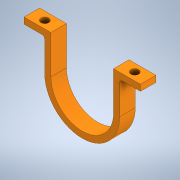
# Autodesk Inventor part: motor_support_v2
Saved by Autodesk Inventor 2020.3 (Build 243373000, 373)
## iProperties
Created: 2020-06-21
Part Number: motor_support_v2
Material: PET Plastic
Document SubType Name: Modeling
Designer: Devin
Density: 1.541 g/cm^3
Appearance: Orange
Author: Devin
Autodesk Inventor part; units mm, degrees
ref_plane "YZ Plane" through (0, 0, 0) normal (1, 0, 0) x (0, 1, 0)
ref_plane "XZ Plane" through (0, 0, 0) normal (0, 1, 0) x (-1, 0, 0)
ref_plane "XY Plane" through (0, 0, 0) normal (0, 0, 1) x (1, 0, 0)
sketch "Sketch1" plane through (0, 0, 0) normal (0, 0, 1) x (1, 0, 0)
  line L0 (-22.529, 12.5) -> (-14.529, 12.5)
  line L1 (22.5896, 12.5) -> (14.571, 12.5)
  line L2 (12.171, 14.9) -> (22.5896, 14.9)
  line L3 (22.5896, 14.9) -> (22.5896, 12.5)
  line L4 (-12.129, 14.9) -> (-22.529, 14.9)
  line L5 (-22.529, 14.9) -> (-22.529, 12.5)
  line L6 (-12.129, 0) -> (-12.129, 14.9)
  line L7 (12.171, 0) -> (12.171, 14.9)
  arc A0 (-12.129, 0) -> (12.171, 0) centre (0.021, 0) ccw
  arc A1 (-14.529, 0) -> (14.571, 0) centre (0.021, 0) ccw
  line L8 (-14.529, 12.5) -> (-14.529, -0.0004)
  line L9 (14.571, 12.5) -> (14.571, 0)
  point P0 (0, 0)
  point P1 (14.6524, 0.7379)
  dimension "d34" = 14.9
  dimension "d35" = 14.9
  dimension "d38" = 2.4
  dimension "d39" = 2.4
  dimension "d46" = 24.3
  dimension "d47" = 2.4
  dimension "d48" = 2.4
  constraints: 20 end point, 5 point on circle, 4 perpendicular, 2 centre point, 2 horizontal, 2 point on line, 2 vertical
  measures "d34" distance from line of L2 point (0, 0)
  measures "d35" distance from line of L4 point (0, 0)
  measures "d38" distance between parallel lines of L2 L1
  measures "d39" distance between parallel lines of L0 L4
  measures "d46" diameter of A0
  measures "d47" radial gap between concentric circles of A0 A1
  measures "d48" distance between parallel lines of L9 L7
extrude "Extrusion5" add sketch "Sketch1" along normal blind 6
fillet "Fillet7" radius 1 1 edges at (14.571, 12.5, 3)
fillet "Fillet8" radius 1 1 edges at (-14.529, 12.5, 3)
sketch "Sketch5" plane through (12.171, 14.9, 0) normal (0, 1, 0) x (1, 0, 0)
  line L0 (10.4185, 0) -> (10.4185, -6)
  line L1 (3.4, 0) -> (10.4185, 0) projected
  circle A0 centre (5.2093, -3) radius 1.5
  circle A1 centre (-29.5299, -3.1217) radius 1.5
  point P0 (-12.171, 0)
  dimension "d54" = 3
  constraints: 2 centre point, 2 end point
  measures "d54" diameter of A0
extrude "Extrusion6" cut sketch "Sketch5" against normal blind 10
body "Solid3"
